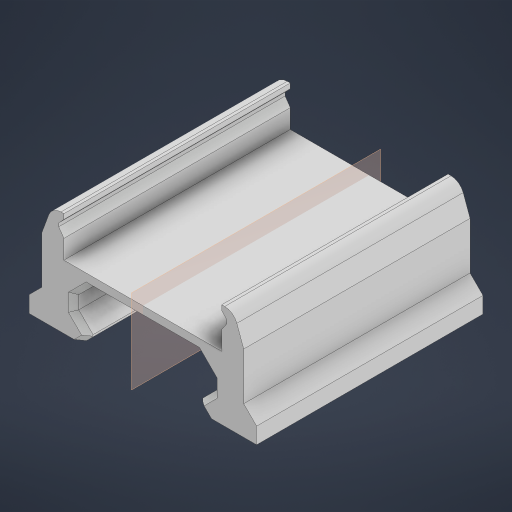
# Autodesk Inventor part: Rail clamp
Saved by Autodesk Inventor 2023 (Build 270158000, 158)
## iProperties
Created: 2023-10-16
Part Number: Rail clamp
Material: Generic
Document SubType Name: Modeling
Designer: nick_
Density: 1 g/cm^3
Appearance: Default
Author: nick_
Autodesk Inventor part; units mm, degrees
ref_plane "YZ Plane" through (0, 0, 0) normal (1, 0, 0) x (0, 1, 0)
ref_plane "XZ Plane" through (0, 0, 0) normal (0, 1, 0) x (-1, 0, 0)
ref_plane "XY Plane" through (0, 0, 0) normal (0, 0, 1) x (1, 0, 0)
sketch "Sketch1" plane through (0, 0, 0) normal (0, 0, 1) x (1, 0, 0)
  line L0 (6.1935, -6.1609) -> (-18.8065, -6.1609) construction
  line L1 (6.1935, -3.1609) -> (6.1935, -6.1609) construction
  line L2 (2.0882, -3.1609) -> (6.1935, -3.1609) construction
  line L3 (2.0882, -0.2145) -> (2.0882, -3.1609) construction
  line L4 (4.298, 1.9953) -> (2.0882, -0.2145) construction
  line L5 (4.298, 3.9511) -> (4.298, 1.9953) construction
  line L6 (2.0882, 6.1609) -> (4.298, 3.9511) construction
  line L7 (2.0882, 6.1609) -> (-14.7012, 6.1609) construction
  line L8 (-14.7012, 6.1609) -> (-16.911, 3.9511) construction
  line L9 (-16.911, 3.9511) -> (-16.911, 1.9953) construction
  line L10 (-16.911, 1.9953) -> (-14.7012, -0.2145) construction
  line L11 (-14.7012, -0.2145) -> (-14.7012, -3.1609) construction
  line L12 (-14.7012, -3.1609) -> (-18.8065, -3.1609) construction
  line L13 (-18.8065, -3.1609) -> (-18.8065, -6.1609) construction
  line L14 (2.1882, -3.0609) -> (6.2935, -3.0609)
  line L15 (6.2935, -3.0609) -> (6.2935, -6.2609)
  line L16 (6.2935, -6.2609) -> (-18.9065, -6.2609)
  line L17 (-18.9065, -6.2609) -> (-18.9065, -3.0609)
  line L18 (-18.9065, -3.0609) -> (-14.8012, -3.0609)
  line L19 (-14.8012, -3.0609) -> (-14.8012, -0.2559)
  line L20 (-14.8012, -0.2559) -> (-17.011, 1.9539)
  line L21 (-17.011, 1.9539) -> (-17.011, 3.9925)
  line L22 (-17.011, 3.9925) -> (-14.7427, 6.2609)
  line L23 (-14.7427, 6.2609) -> (2.1296, 6.2609)
  line L24 (2.1296, 6.2609) -> (4.398, 3.9925)
  line L25 (4.398, 3.9925) -> (4.398, 1.9539)
  line L26 (4.398, 1.9539) -> (2.1882, -0.2559)
  line L27 (2.1882, -0.2559) -> (2.1882, -3.0609)
  line L28 (11.2935, 0.9391) -> (9.2935, 0.9391)
  line L29 (9.2935, 0.9391) -> (9.2935, 10.2609)
  line L30 (-21.9065, 10.2609) -> (-21.9065, 0.9391)
  line L31 (-21.9065, 0.9391) -> (-23.9065, 0.9391)
  line L32 (-23.9065, 0.9391) -> (-23.9065, -1.5609)
  line L33 (11.2935, -1.5609) -> (11.2935, 0.9391)
  line L34 (2.1882, -1.5609) -> (11.2935, -1.5609)
  line L35 (-14.8012, -1.5609) -> (-23.9065, -1.5609)
  line L36 (-21.9065, 10.2609) -> (9.2935, 10.2609)
  point P0 (0, 0)
  point P1 (-21.9065, 6.0636)
  point P2 (6.7408, -1.5609)
  point P3 (-19.3539, -1.5609)
  point P4 (-6.3065, 10.2609)
  point P5 (-6.3065, -6.2609)
  point P6 (-22.9065, 0.9391)
  point P7 (10.2935, 0.9391)
  dimension "d0" = 0.1
  dimension "d1" = 5
  dimension "d2" = 1.5
  dimension "d5" = 5
  dimension "d44" = 4
  dimension "d45" = 2
  dimension "d46" = 2.5
  constraints: 46 end point, 6 midpoint, 4 perpendicular, 3 point on line, 2 horizontal alignment, 1 collinear, 1 horizontal, 1 vertical, 1 vertical alignment, 13 other
  measures "d0" distance between parallel lines of L3 L27
  measures "d1" distance between parallel lines of L33 L15
  measures "d2" distance between parallel lines of L34 L14
  measures "d5" distance between parallel lines of L32 L17
  measures "d44" distance between parallel lines of L36 L23
  measures "d45" distance of L28.start L28.end
  measures "d46" distance from line of L35 point (-22.907, 0.939)
extrude "Extrusion1" add sketch "Sketch1" against normal blind 35 contours L27 L26 L25 L24 L23 L22 L21 L20 L19 L35 L32 L31 L30 L36 L29 L28 L33 L34
ref_plane "Work Plane2" through (-6.3065, 0.9391, 0) normal (1, 0, 0) x (0, 0, -1)
chamfer "Chamfer1" distance 1 angle 45 2 edges at (-14.8012, -1.5609, -17.5) (2.1882, -1.5609, -17.5)
sketch "Sketch3" plane through (0, 0, -35) normal (0, 0, -1) x (-1, 0, 0)
  line L0 (18.9065, 11.7609) -> (-6.2935, 11.7609) construction
  line L1 (-6.2935, 11.7609) -> (-6.2935, 13.2909) construction
  line L2 (18.9065, 13.2909) -> (-6.2935, 13.2909) construction
  line L3 (18.9065, 11.7609) -> (18.9065, 13.2909) construction
  line L4 (-2.1882, -0.5609) -> (-3.1882, -1.5609) construction
  line L5 (-2.1882, -0.5609) -> (-2.1882, -0.2559) construction
  line L6 (-2.1882, -0.2559) -> (-4.398, 1.9539) construction
  line L7 (-4.398, 1.9539) -> (-4.398, 3.9925) construction
  line L8 (-4.398, 3.9925) -> (-2.1296, 6.2609) construction
  line L9 (-2.1296, 6.2609) -> (14.7427, 6.2609) construction
  line L10 (14.7427, 6.2609) -> (17.011, 3.9925) construction
  line L11 (17.011, 3.9925) -> (17.011, 1.9539) construction
  line L12 (17.011, 1.9539) -> (14.8012, -0.2559) construction
  line L13 (14.8012, -0.2559) -> (14.8012, -0.5609) construction
  line L14 (15.8012, -1.5609) -> (14.8012, -0.5609) construction
  line L15 (15.8012, -1.5609) -> (23.9065, -1.5609) construction
  line L16 (23.9065, -1.5609) -> (23.9065, 0.9391) construction
  line L17 (23.9065, 0.9391) -> (21.9065, 0.9391) construction
  line L18 (21.9065, 0.9391) -> (21.9065, 10.2609) construction
  line L19 (21.9065, 10.2609) -> (-9.2935, 10.2609) construction
  line L20 (-9.2935, 10.2609) -> (-9.2935, 0.9391) construction
  line L21 (-9.2935, 0.9391) -> (-11.2935, 0.9391) construction
  line L22 (-11.2935, 0.9391) -> (-11.2935, -1.5609) construction
  line L23 (-11.2935, -1.5609) -> (-3.1882, -1.5609) construction
  line L24 (-2.0533, 10.2609) -> (-2.0533, 8.2609)
  line L25 (-9.2935, 10.2609) -> (21.9065, 10.2609) projected
  line L26 (-3.1882, -1.5609) -> (-2.1882, -0.5609) construction
  line L27 (-3.1882, -1.5609) -> (-11.2935, -1.5609) construction
  line L28 (-11.2935, -1.5609) -> (-11.2935, 0.9391) construction
  line L29 (-11.2935, 0.9391) -> (-9.2935, 0.9391) construction
  line L30 (-9.2935, 0.9391) -> (-9.2935, 10.2609) construction
  line L31 (-9.2935, 10.2609) -> (21.9065, 10.2609) construction
  line L32 (21.9065, 10.2609) -> (21.9065, 0.9391) construction
  line L33 (21.9065, 0.9391) -> (23.9065, 0.9391) construction
  line L34 (23.9065, 0.9391) -> (23.9065, -1.5609) construction
  line L35 (23.9065, -1.5609) -> (15.8012, -1.5609) construction
  line L36 (14.8012, -0.5609) -> (15.8012, -1.5609) construction
  line L37 (14.8012, -0.5609) -> (14.8012, -0.2559) construction
  line L38 (14.8012, -0.2559) -> (17.011, 1.9539) construction
  line L39 (17.011, 1.9539) -> (17.011, 3.9925) construction
  line L40 (17.011, 3.9925) -> (14.7427, 6.2609) construction
  line L41 (14.7427, 6.2609) -> (-2.1296, 6.2609) construction
  line L42 (-2.1296, 6.2609) -> (-4.398, 3.9925) construction
  line L43 (-4.398, 3.9925) -> (-4.398, 1.9539) construction
  line L44 (-4.398, 1.9539) -> (-2.1882, -0.2559) construction
  line L45 (-2.1882, -0.2559) -> (-2.1882, -0.5609) construction
  line L46 (21.9065, 10.2609) -> (20.3669, 14.4909)
  line L47 (20.3669, 14.4909) -> (18.5065, 14.4909)
  line L48 (18.5065, 14.4909) -> (18.5065, 13.7199)
  line L49 (18.5065, 13.7199) -> (19.3065, 12.8619)
  line L50 (19.3065, 12.8619) -> (19.3065, 12.3385)
  line L51 (19.3065, 12.3385) -> (18.5065, 11.1833)
  line L52 (18.5065, 11.1833) -> (18.5065, 10.2609)
  point P0 (0, 0)
  point P1 (18.5065, 14.1054)
  point P2 (18.5065, 10.7221)
  dimension "d48" = 0.4
  dimension "d49" = 1.2
  dimension "d50" = 70
  constraints: 16 end point, 4 midpoint, 2 perpendicular, 2 point on line, 1 horizontal, 1 parallel, 1 vertical, 1 vertical alignment
  measures "d48" distance between parallel lines of L3 L50
  measures "d49" distance between parallel lines of L2 L47
  measures "d50" angle of L25 L46
chamfer "Chamfer2" distance 0.8 angle 45 21 edges at (4.398, 2.9732, 0) (3.2931, 0.849, 0) (2.1882, -0.4084, 0) (3.2638, 5.1267, 0) (-6.3065, 6.2609, 0) (-15.8768, 5.1267, 0) (-17.011, 2.9732, 0) (-15.9061, 0.849, 0) (-15.3012, -1.0609, 0) (2.6882, -1.0609, 0) (3.2638, 5.1267, -35) (4.398, 2.9732, -35) (3.2931, 0.849, -35) (2.1882, -0.4084, -35) (-15.3012, -1.0609, -35) (-14.8012, -0.4084, -35) (-15.9061, 0.849, -35) (-17.011, 2.9732, -35) (-15.8768, 5.1267, -35) (-6.3065, 6.2609, -35) (2.6882, -1.0609, -35)
extrude "Extrusion5" add sketch "Sketch3" against normal up to surface (35 mm away)
mirror "Mirror3" about plane through (-6.3065, 0.9391, 0) normal (1, 0, 0) of "Extrusion5"
fillet "Fillet3" radius 2 2 edges at (-20.3669, 14.4909, -17.5) (7.7539, 14.4909, -17.5)
sketch "Sketch6" plane through (0, 0, 0) normal (0, 0, 1) x (1, 0, 0)
  arc A0 (8.2328, 13.1749) -> (6.3535, 14.4909) centre (6.3535, 12.4909) ccw construction
  line L0 (6.3535, 14.4909) -> (5.8935, 14.4909) construction
  line L1 (5.8935, 14.4909) -> (5.8935, 13.7199) construction
  line L2 (5.8935, 13.7199) -> (6.6935, 12.8619) construction
  line L3 (6.6935, 12.8619) -> (6.6935, 12.3385) construction
  line L4 (6.6935, 12.3385) -> (5.8935, 11.1833) construction
  line L5 (5.8935, 11.1833) -> (5.8935, 10.2609) construction
  line L6 (5.8935, 10.2609) -> (-18.5065, 10.2609) construction
  line L7 (-18.5065, 11.1833) -> (-18.5065, 10.2609) construction
  line L8 (-19.3065, 12.3385) -> (-18.5065, 11.1833) construction
  line L9 (-19.3065, 12.8619) -> (-19.3065, 12.3385) construction
  line L10 (-18.5065, 13.7199) -> (-19.3065, 12.8619) construction
  line L11 (-18.5065, 14.4909) -> (-18.5065, 13.7199) construction
  line L12 (-18.9665, 14.4909) -> (-18.5065, 14.4909) construction
  arc A1 (-18.9665, 14.4909) -> (-20.8459, 13.1749) centre (-18.9665, 12.4909) ccw construction
  line L13 (-21.9065, 10.2609) -> (-20.8459, 13.1749) construction
  line L14 (-21.9065, 10.2609) -> (-21.9065, 0.9391) construction
  line L15 (-21.9065, 0.9391) -> (-23.9065, 0.9391) construction
  line L16 (-23.9065, 0.9391) -> (-23.9065, -1.5609) construction
  line L17 (-23.9065, -1.5609) -> (-16.9326, -1.5609) construction
  line L18 (-15.7801, -0.4084) -> (-16.9326, -1.5609) construction
  line L19 (-17.811, 1.6225) -> (-15.7801, -0.4084) construction
  line L20 (-17.811, 4.3239) -> (-17.811, 1.6225) construction
  line L21 (-15.074, 7.0609) -> (-17.811, 4.3239) construction
  line L22 (2.461, 7.0609) -> (-15.074, 7.0609) construction
  line L23 (5.198, 4.3239) -> (2.461, 7.0609) construction
  line L24 (5.198, 1.6225) -> (5.198, 4.3239) construction
  line L25 (3.167, -0.4084) -> (5.198, 1.6225) construction
  line L26 (4.3195, -1.5609) -> (3.167, -0.4084) construction
  line L27 (4.3195, -1.5609) -> (11.2935, -1.5609) construction
  line L28 (11.2935, -1.5609) -> (11.2935, 0.9391) construction
  line L29 (11.2935, 0.9391) -> (9.2935, 0.9391) construction
  line L30 (9.2935, 0.9391) -> (9.2935, 10.2609) construction
  line L31 (9.2935, 10.2609) -> (8.2328, 13.1749) construction
  line L32 (-18.5065, 11.1833) -> (-18.5065, 10.2609) projected
  line L33 (-18.5065, 10.2609) -> (5.8935, 10.2609)
  line L34 (5.8935, 10.2609) -> (5.8935, 8.2609)
  line L35 (5.8935, 8.2609) -> (-18.5065, 8.2609)
  line L36 (-18.5065, 8.2609) -> (-18.5065, 10.2609)
  point P0 (0, 0)
  dimension "d54" = 2
  constraints: 8 end point, 2 parallel, 1 horizontal, 1 perpendicular
  measures "d54" distance of L33.end L34.end
extrude "Extrusion6" cut sketch "Sketch6" against normal through all
chamfer "Chamfer4" distance 2 angle 45 2 edges at (9.2935, 0.9391, -17.5) (-21.9065, 0.9391, -17.5)
equation "\"d5\" = d1"
body "Solid1"
